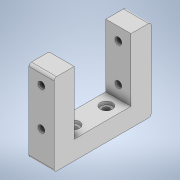
# Autodesk Inventor part: LowerJaw
Saved by Autodesk Inventor 2022 (Build 260153000, 153)
## iProperties
Created: 2021-11-02
Part Number: LowerJaw
Material: Genérico
Document SubType Name: Modeling
Designer: JK
Density: 1 g/cm^3
Appearance: Valor por defecto
Author: JK
Autodesk Inventor part; units mm, degrees
ref_plane "YZ Plane" through (0, 0, 0) normal (1, 0, 0) x (0, 1, 0)
ref_plane "XZ Plane" through (0, 0, 0) normal (0, 1, 0) x (-1, 0, 0)
ref_plane "XY Plane" through (0, 0, 0) normal (0, 0, 1) x (1, 0, 0)
sketch "Boceto1" plane through (0, 0, 0) normal (0, 1, 0) x (-1, 0, 0)
  line L0 (-6.45, 25.5) -> (6.45, 25.5)
  line L1 (6.45, 25.5) -> (6.45, -25.5)
  line L2 (6.45, -25.5) -> (-6.45, -25.5)
  line L3 (-6.45, -25.5) -> (-6.45, 25.5)
  line L4 (-6.45, 25.5) -> (6.45, -25.5) construction
  line L5 (6.45, 25.5) -> (-6.45, -25.5) construction
  circle A0 centre (0, 0) radius 3.5
  dimension "d0" = 7
  dimension "d1" = 51
  dimension "d2" = 12.9
  constraints: 12 end point, 2 midpoint, 2 parallel, 1 centre point, 1 coincident, 1 horizontal, 1 perpendicular
  measures "d0" diameter of A0
  measures "d1" distance of L0.end L1.end
  measures "d2" distance of L1.end L2.end
extrude "Extrusión1" add sketch "Boceto1" along normal blind 10
sketch "Boceto2" plane through (0, 10, 0) normal (0, 1, 0) x (1, 0, 0)
  circle A0 centre (0, 0) radius 6
  dimension "d5" = 12
  constraints: 1 centre point, 1 coincident
  measures "d5" diameter of A0
extrude "Extrusión2" cut sketch "Boceto2" against normal blind 6
sketch "Boceto3" plane through (0, 10, 0) normal (0, 1, 0) x (1, 0, 0)
  circle A0 centre (0, 0) radius 6 projected
  line L0 (6.45, 25.5) -> (-6.45, 25.5) projected
  line L1 (-6.45, 25.5) -> (-6.45, -25.5) projected
  line L2 (-6.45, -25.5) -> (6.45, -25.5) projected
  line L3 (6.45, -25.5) -> (6.45, 25.5) projected
  line L4 (10, -38.575) -> (-10, -38.575)
  line L5 (-10, -38.575) -> (-10, 38.575)
  line L6 (-10, 38.575) -> (10, 38.575)
  line L7 (10, 38.575) -> (10, -38.575)
  line L8 (10, -38.575) -> (-10, 38.575) construction
  line L9 (-10, -38.575) -> (10, 38.575) construction
  dimension "d21" = 20
  dimension "d22" = 77.15
  constraints: 12 end point, 2 midpoint, 2 parallel, 1 horizontal, 1 perpendicular
  measures "d21" distance of L5.end L6.end
  measures "d22" distance of L6.end L4.start
extrude "Extrusión3" add sketch "Boceto3" against normal blind 15 contours L4 L5 L6 L7
sketch "Boceto4" plane through (0, 10, 0) normal (0, 1, 0) x (1, 0, 0)
  line L0 (10, -38.575) -> (-10, -38.575) projected
  line L1 (10, -38.575) -> (10, 38.575) projected
  line L2 (-10, -38.575) -> (10, -38.575)
  line L3 (10, -38.575) -> (10, -22.575)
  line L4 (10, -22.575) -> (-10, -22.575)
  line L5 (-10, -22.575) -> (-10, -38.575)
  line L6 (10, 38.575) -> (-10, 38.575) projected
  line L7 (-10, 38.575) -> (10, 38.575)
  line L8 (10, 38.575) -> (10, 22.575)
  line L9 (10, 22.575) -> (-10, 22.575)
  line L10 (-10, 22.575) -> (-10, 38.575)
  point P0 (0, 0)
  point P1 (10, 22.575)
  dimension "d12" = 16
  dimension "d13" = 16
  constraints: 16 end point, 4 parallel, 2 horizontal, 2 perpendicular, 2 point on line
  measures "d12" distance between parallel lines of L4 L0
  measures "d13" distance between parallel lines of L6 L9
extrude "Extrusión4" add sketch "Boceto4" along normal blind 50
sketch "Boceto5" plane through (-10, -5, 38.575) normal (0, 0, 1) x (1, 0, 0)
  circle A0 centre (10, 55) radius 2.7
  circle A1 centre (10, 25) radius 2.6954
  line L0 (0, 65) -> (20, 65) projected
  point P0 (10, 5)
  point P1 (20, 15)
  dimension "d16" = 5.4
  dimension "d17" = 10
  dimension "d18" = 10
  constraints: 2 centre point, 2 vertical alignment
  measures "d16" diameter of A0
  measures "d17" distance from line of L0 A0.centre
  measures "d18" horizontal distance of point (20, 15) A1.centre
extrude "Extrusión5" cut sketch "Boceto5" against normal through all
sketch "Boceto6" plane through (0, 10, 0) normal (0, 1, 0) x (1, 0, 0)
  circle A0 centre (0, 0) radius 6 projected
extrude "Extrusión6" add sketch "Boceto6" against normal up to surface (10 mm away)
sketch "Boceto7" plane through (0, -5, 0) normal (0, -1, 0) x (1, 0, 0)
  line L0 (-10, -38.575) -> (10, -38.575) projected
  line L1 (10, -38.575) -> (10, 38.575) projected
  line L2 (10, 38.575) -> (-10, 38.575) projected
  line L3 (-10, 38.575) -> (-10, -38.575) projected
  line L4 (6.45, 25.5) -> (6.45, -25.5) projected
  line L5 (6.45, -25.5) -> (-6.45, -25.5) projected
  line L6 (-6.45, -25.5) -> (-6.45, 25.5) projected
  line L7 (-6.45, 25.5) -> (6.45, 25.5) projected
  line L8 (6.45, -25.5) -> (-6.45, -25.5) projected
  line L9 (6.45, 25.5) -> (6.45, -25.5) projected
  line L10 (-6.45, 25.5) -> (6.45, 25.5) projected
  line L11 (-6.45, -25.5) -> (-6.45, 25.5) projected
  point P0 (0, 0)
extrude "Extrusión7" add sketch "Boceto7" against normal up to surface (5 mm away) contours L4 L5 L6 L7
sketch "Boceto8" plane through (0, 10, 0) normal (0, 1, 0) x (1, 0, 0)
  circle A0 centre (0, -13) radius 2.7
  circle A1 centre (0, 13) radius 2.7
  point P0 (0, 0)
  dimension "d27" = 5.4
  dimension "d28" = 13
  dimension "d29" = 13
  constraints: 2 centre point, 1 equal radius
  measures "d27" diameter of A0
  measures "d28" distance of point (0, 0) A0.centre
  measures "d29" distance of point (0, 0) A1.centre
extrude "Extrusión8" cut sketch "Boceto8" against normal through all
sketch "Boceto9" plane through (0, 10, 0) normal (0, 1, 0) x (1, 0, 0)
  circle A0 centre (0, -13) radius 2.7 projected
  circle A1 centre (0, -13) radius 4.75
  circle A2 centre (0, 13) radius 2.7 projected
  circle A3 centre (0, 13) radius 4.75
  point P0 (0, 0)
  dimension "d32" = 9.5
  dimension "d33" = 9.5
  constraints: 2 centre point, 2 coincident
  measures "d32" diameter of A1
  measures "d33" diameter of A3
extrude "Extrusión9" cut sketch "Boceto9" against normal blind 2.5
fillet "Empalme1" radius 2 4 edges at (0, -5, 38.575) (0, 60, 38.575) (0, 60, -38.575) (0, -5, -38.575)
